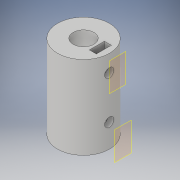
# Autodesk Inventor part: radianprintercoupler
Saved by Autodesk Inventor 2019 (Build 230136000, 136)
## iProperties
Created: 2019-09-15
Part Number: radianprintercoupler
Material: Generic
Document SubType Name: Modeling
Designer: rob
Density: 1 g/cm^3
Appearance: Default
Author: rob
Autodesk Inventor part; units mm, degrees
ref_plane "YZ Plane" through (0, 0, 0) normal (1, 0, 0) x (0, 1, 0)
ref_plane "XZ Plane" through (0, 0, 0) normal (0, 1, 0) x (-1, 0, 0)
ref_plane "XY Plane" through (0, 0, 0) normal (0, 0, 1) x (1, 0, 0)
sketch "Sketch1" plane through (0, 0, 0) normal (0, 1, 0) x (-1, 0, 0)
  circle A0 centre (0, 0) radius 4
  circle A1 centre (0, 0) radius 10
  dimension "d0" = 8
  dimension "d1" = 20
  constraints: 2 centre point, 2 coincident
  measures "d0" diameter of A0
  measures "d1" diameter of A1
extrude "Extrusion1" add sketch "Sketch1" along normal blind 16
sketch "Sketch2" plane through (0, 16, 0) normal (0, 1, 0) x (1, 0, 0)
  line L0 (5, -2.75) -> (7.7, -2.75)
  line L1 (7.7, -2.75) -> (7.7, 3.05)
  line L2 (7.7, 3.05) -> (5, 3.05)
  line L3 (5, 3.05) -> (5, -2.75)
  point P0 (0, 0)
  dimension "d4" = 2.7
  dimension "d5" = 5.8
  dimension "d6" = 2.75
  dimension "d7" = 5
  constraints: 8 end point, 2 parallel, 1 horizontal, 1 perpendicular
  measures "d4" distance of L2.end L1.end
  measures "d5" distance of L1.end L0.end
  measures "d6" distance from line of point (0, 0) L0
  measures "d7" distance from line of point (0, 0) L3
extrude "Extrusion2" cut sketch "Sketch2" against normal blind 10
ref_plane "Work Plane1" through (13, 16, 2.75) normal (1, 0, 0) x (0, 0, -1)
sketch "Sketch3" plane through (13, 16, 2.75) normal (1, 0, 0) x (0, 0, -1)
  circle A0 centre (2.75, -6.5) radius 1.75
  line L0 (5.8, -10) -> (0, -10) projected
  point P0 (2.75, -16)
  dimension "d11" = 3.5
  dimension "d12" = 3.5
  constraints: 1 centre point
  measures "d11" diameter of A0
  measures "d12" distance from line of A0.centre L0
extrude "Extrusion3" cut sketch "Sketch3" against normal blind 10
sketch "Sketch4" plane through (0, 0, 0) normal (0, -1, 0) x (1, 0, 0)
  circle A0 centre (0, 0) radius 4
  circle A1 centre (0, 0) radius 10
  constraints: 2 centre point, 2 coincident
extrude "Extrusion4" add sketch "Sketch4" along normal blind 16
sketch "Sketch5" plane through (0, -16, 0) normal (0, -1, 0) x (1, 0, 0)
  line L0 (5, 2.75) -> (5, -3.05) projected
  line L1 (7.7, -3.05) -> (7.7, 2.75) projected
  line L2 (5, 2.75) -> (7.7, 2.75)
  line L3 (7.7, 2.75) -> (7.7, -3.05)
  line L4 (7.7, -3.05) -> (5, -3.05)
  line L5 (5, -3.05) -> (5, 2.75)
  point P0 (0, 0)
  constraints: 8 end point, 2 parallel, 1 horizontal, 1 perpendicular
extrude "Extrusion5" cut sketch "Sketch5" against normal blind 12
ref_plane "Work Plane2" through (15, -16, 2.75) normal (1, 0, 0) x (0, 0, -1)
sketch "Sketch6" plane through (15, -16, 2.75) normal (1, 0, 0) x (0, 0, -1)
  circle A0 centre (2.75, 9) radius 1.75
  line L0 (-7.25, 0) -> (12.75, 0) projected
  point P0 (2.75, 16)
  dimension "d20" = 3.5
  dimension "d34" = 9
  constraints: 1 centre point
  measures "d20" diameter of A0
  measures "d34" distance from line of L0 A0.centre
extrude "Extrusion6" cut sketch "Sketch6" against normal blind 15
sketch "Sketch7" plane through (0, -16, 0) normal (0, -1, 0) x (1, 0, 0)
  circle A0 centre (0, 0) radius 4 projected
  line L0 (-3.7528, -6.5) -> (-7.5056, 0)
  line L1 (7.5056, 0) -> (3.7528, -6.5)
  line L2 (-3.7528, 6.5) -> (3.7528, 6.5)
  line L3 (-7.5056, 0) -> (-3.7528, 6.5)
  line L4 (3.7528, -6.5) -> (-3.7528, -6.5)
  line L5 (3.7528, 6.5) -> (7.5056, 0)
  circle A1 centre (0, 0) radius 4
  constraints: 12 end point, 2 coincident, 1 centre point, 1 concentric, 1 horizontal, 1 parallel, 2 other
extrude "Extrusion7" cut sketch "Sketch7" against normal blind 7
body "Solid1"
